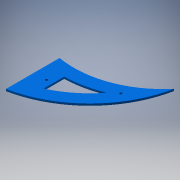
# Autodesk Inventor part: landing-gear-claws
Saved by Autodesk Inventor 2016 (Build 200138000, 138)
## iProperties
Created: 2015-01-28
Part Number: landing-gear-claws
Material: ABS Plastic
Document SubType Name: Modeling
Designer: Vasanth
Density: 1.06 g/cm^3
Appearance: Smooth - White
Mass: 14.4939 g
Surface Area: 147.925 cm^2
Volume: 13.6735 cm^3
Author: Vasanth
Autodesk Inventor part; units mm, degrees
ref_plane "YZ Plane" through (0, 0, 0) normal (1, 0, 0) x (0, 1, 0)
ref_plane "XZ Plane" through (0, 0, 0) normal (0, 1, 0) x (-1, 0, 0)
ref_plane "XY Plane" through (0, 0, 0) normal (0, 0, 1) x (1, 0, 0)
sketch "Sketch12" plane through (0, 0, 0) normal (0, 1, 0) x (-1, 0, 0)
  arc A0 (-17.9101, 19.3197) -> (-99.957, -10.5429) centre (-33.0718, -66.6663) ccw
  arc A1 (-36.0097, 32.8266) -> (-70.4306, 25.593) centre (-33.0718, -66.6663) ccw
  circle A2 centre (-30.1338, 44.1595) radius 1.016
  line L0 (-36.0097, 32.8266) -> (-36.0097, 53.0201)
  arc A3 (-36.0097, 53.0201) -> (-70.4306, 25.593) centre (2.8014, -31.0003) ccw
  line L1 (-17.9101, 19.3197) -> (-17.9101, 71.7072)
  arc A4 (-17.9101, 71.7072) -> (-99.957, -10.5429) centre (2.8014, -31.0003) ccw
  circle A5 centre (-30.1338, 44.1595) radius 1.2065
  circle A6 centre (-77.8759, 19.3514) radius 1.2065
  constraints: 8 point on circle, 7 centre point, 4 end point, 2 vertical, 1 coincident
extrude "Extrusion13" add sketch "Sketch12" along normal blind 1.905 contours A0 A4 L1
body "Solid2"
